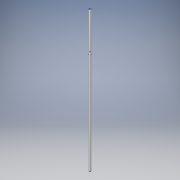
# Autodesk Inventor part: tubo_instrumentação_2500mm
Saved by Autodesk Inventor 2019.4 (Build 234330000, 330)
## iProperties
Created: 2021-02-17
Part Number: tubo_instrumentação_2500mm
Material: Alumínio 6061
Document SubType Name: Modeling
Designer: Lattes
Density: 2.7 g/cm^3
Appearance: Alumínio - Plano
Author: Lattes
Autodesk Inventor part; units mm, degrees
ref_plane "XZ Plane" through (0, 0, 0) normal (0, 1, 0) x (-1, 0, 0)
sketch "Esboço1" plane through (0, 0, 0) normal (0, 1, 0) x (-1, 0, 0)
  circle A0 centre (0, 0) radius 14.5
  circle A1 centre (0, 0) radius 16
  dimension "d0" = 29
  dimension "d1" = 32
  constraints: 2 centre point, 2 coincident
  measures "d0" diameter of A0
  measures "d1" diameter of A1
extrude "Extrusão1" add sketch "Esboço1" along normal blind 2500
ref_plane "Plano de trabalho2" through (-16, 0, 0) normal (1, 0, 0) x (0, 1, 0)
sketch "Esboço2" plane through (-16, 0, 0) normal (1, 0, 0) x (0, 1, 0)
  line L0 (2500, -16) -> (2500, 16) projected
  line L1 (2500, 0) -> (1900, 0)
  circle A0 centre (1900, 0) radius 1.75
  circle A1 centre (1900, 0) radius 3
  point P0 (0, 0)
  dimension "d6" = 600
  dimension "d7" = 3.5
  dimension "d8" = 6
  constraints: 2 centre point, 2 coincident, 2 end point, 1 horizontal, 1 midpoint
  measures "d6" distance of L1.start L1.end
  measures "d7" diameter of A0
  measures "d8" diameter of A1
extrude "Extrusão2" add sketch "Esboço2" along normal blind 0.5
sketch "Esboço3" plane through (-16, 0, 0) normal (-1, 0, 0) x (0, 0, 1)
  arc A0 (0, 1898.25) -> (0, 1901.75) centre (0, 1900) ccw projected
  circle A1 centre (0, 1900) radius 1.75
  point P0 (0, 0)
  constraints: 1 centre point, 1 coincident
extrude "Extrusão3" cut sketch "Esboço3" against normal blind 5
sketch "Esboço4" plane through (-16, 0, 0) normal (1, 0, 0) x (0, 1, 0)
  line L0 (2500, 14.5) -> (2500, -14.5) projected
  line L1 (2500, 0) -> (1840, 0)
  line L2 (1840, 0) -> (1470, 0)
  circle A0 centre (1470, 0) radius 2
  circle A1 centre (1470, 0) radius 3
  line L3 (1470, 0) -> (1430, 0)
  line L4 (1470, 0) -> (1510, 0) construction
  point P0 (0, 0)
  dimension "d13" = 660
  dimension "d14" = 370
  dimension "d15" = 4
  dimension "d16" = 6
  dimension "d21" = 40
  dimension "d22" = 180
  constraints: 8 end point, 3 horizontal, 2 centre point, 2 coincident, 1 collinear, 1 midpoint, 1 point on line
  measures "d13" distance of L1.start L1.end
  measures "d14" distance of L1.end L2.end
  measures "d15" diameter of A0
  measures "d16" diameter of A1
  measures "d21" distance of L3.start L3.end
  measures "d22" angle of L3 L4
extrude "Extrusão4" add sketch "Esboço4" along normal blind 0.5 contours A1 L3 A0 L2 | L2 A0 L3 A1
sketch "Esboço5" plane through (-16, 0, 0) normal (-1, 0, 0) x (0, 0, 1)
  arc A0 (0, 1472) -> (0, 1468) centre (0, 1470) ccw projected
  circle A1 centre (0, 1470) radius 2.1
  point P0 (0, 0)
  point P1 (0, 1741.75)
  point P2 (0, 1738.25)
  point P3 (0, 1438.25)
  point P4 (0, 1441.75)
  point P5 (0, 1468.25)
  point P6 (0, 1471.75)
  dimension "d107" = 4.2
  constraints: 1 coincident, 3 other
extrude "Extrusão5" cut sketch "Esboço5" against normal blind 10
ref_plane "Plano de trabalho3" through (0, 0, 16) normal (0, 0, 1) x (1, 0, 0)
pattern_circular "Padrão circular3" count 2 over 360 about axis through (0, 0, 0) along (0, 1, 0) of "Extrusão1"
sketch "Esboço19" plane through (0, 2500, 0) normal (0, 1, 0) x (1, 0, 0)
  circle A0 centre (0, 0) radius 16
  line L0 (0, 0) -> (11.3137, 11.3137)
  line L1 (0, 0) -> (16, 0) construction
  line L2 (11.3137, 11.3137) -> (-10.253, -10.253)
  circle A1 centre (0, 0) radius 14.5 projected
  line L3 (0, 0) -> (11.3137, -11.3137)
  line L4 (0, 0) -> (-11.3137, 11.3137)
  circle A2 centre (0, 0) radius 16 projected
  dimension "d77" = 45
  constraints: 10 end point, 3 point on circle, 2 point on line, 1 centre point, 1 coincident, 1 equal length, 1 horizontal, 1 perpendicular, 2 other
  measures "d77" angle of L1 L0
ref_plane "Plano de trabalho4" through (11.3137, 2500, -11.3137) normal (0.7071068, 0, -0.7071068) x (0, 1, 0)
sketch "Esboço20" plane through (11.3137, 2500, -11.3137) normal (0.7071068, 0, -0.7071068) x (0, 1, 0)
  line L0 (0, 14.5) -> (0, -14.5) projected
  line L1 (0, 0) -> (-700, 0)
  circle A0 centre (-700, 0) radius 4.5
  point P0 (-2500, 0)
  dimension "d78" = 700
  dimension "d79" = 9
  constraints: 2 end point, 1 centre point, 1 coincident, 1 horizontal, 1 midpoint
  measures "d78" distance of L1.start L1.end
  measures "d79" diameter of A0
extrude "Extrusão16" add sketch "Esboço20" against normal blind 0.7
pattern_circular "Padrão circular4" count 2 over 360 about axis through (0, 0, 0) along (0, 1, 0) of "Extrusão16"
sketch "Esboço21" plane through (11.3137, 2500, -11.3137) normal (0.7071068, 0, -0.7071068) x (-0.7071068, 0, -0.7071068)
  arc A0 (0, -695.5) -> (0, -704.5) centre (0, -700) ccw projected
  circle A1 centre (0, -700) radius 3.5
  point P0 (0, -2500)
  dimension "d85" = 7
  constraints: 1 centre point, 1 coincident
  measures "d85" diameter of A1
extrude "Extrusão17" cut sketch "Esboço21" against normal blind 50
ref_plane "Plano de trabalho5" through (11.3137, 2500, 11.3137) normal (0.7071068, 0, 0.7071068) x (0, 1, 0)
sketch "Esboço22" plane through (11.3137, 2500, 11.3137) normal (0.7071068, 0, 0.7071068) x (0, 1, 0)
  line L0 (0, 14.5) -> (0, -14.5) projected
  line L1 (0, 0) -> (-700, 0)
  line L2 (-700, 0) -> (-650, 0)
  circle A0 centre (-650, 0) radius 4.5
  point P0 (-2500, 0)
  dimension "d88" = 700
  dimension "d89" = 50
  dimension "d90" = 9
  constraints: 4 end point, 1 centre point, 1 coincident, 1 horizontal, 1 midpoint, 1 point on line
  measures "d88" distance of L1.start L1.end
  measures "d89" distance of L1.end L2.end
  measures "d90" diameter of A0
extrude "Extrusão18" add sketch "Esboço22" against normal blind 0.7
pattern_circular "Padrão circular5" count 2 over 360 about axis through (0, 0, 0) along (0, 1, 0) of "Extrusão18"
sketch "Esboço23" plane through (11.3137, 2500, 11.3137) normal (0.7071068, 0, 0.7071068) x (0.7071068, 0, -0.7071068)
  arc A0 (0, -645.5) -> (0, -654.5) centre (0, -650) ccw projected
  circle A1 centre (0, -650) radius 3.5
  point P0 (0, -2500)
  dimension "d96" = 7
  constraints: 1 centre point, 1 coincident
  measures "d96" diameter of A1
extrude "Extrusão19" cut sketch "Esboço23" against normal blind 50
sketch "Esboço26" plane through (-16, 0, 0) normal (-1, 0, 0) x (0, 0, 1)
  arc A0 (0, 1472.1) -> (0, 1467.9) centre (0, 1470) ccw projected
  circle A1 centre (0, 1470) radius 2
  point P0 (0, 0)
  dimension "d108" = 4
  constraints: 1 centre point, 1 coincident
  measures "d108" diameter of A1
extrude "Extrusão22" cut sketch "Esboço5" against normal blind 10
thread "Rosca2" size "M5x0.8" class "6H" standard "ANSI Metric M Profile" full length
